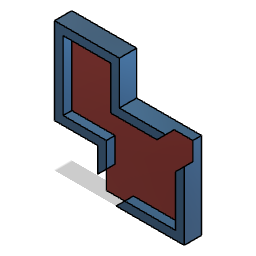
3d07 v122 (Autodesk Fusion 360 design; units mm, degrees)
Autodesk Fusion 360 part; units mm, degrees
sketch "Sketch1" plane through (0, 0, 0) normal (0, 0, 1) x (1, 0, 0)
  line L0 (0, 0) -> (40, 0)
  line L1 (40, 0) -> (40, 40)
  line L2 (40, 40) -> (10, 40)
  line L3 (0, 20) -> (0, 0)
  line L4 (-20, 60) -> (10, 60)
  line L5 (10, 60) -> (10, 40)
  line L6 (0, 20) -> (-20, 20)
  line L7 (-20, 20) -> (-20, 60)
  dimension "d1" = 40
  dimension "d3" = 30
  dimension "d4" = 40
  dimension "d5" = 30
  dimension "d6" = 20
  constraint horizontal L0
  constraint vertical L1
  constraint horizontal L2
  constraint vertical L3
  constraint coincident L0.start L3.end
  constraint horizontal L4
  constraint vertical L5
  constraint horizontal L6
  constraint vertical L7
  measures "d1" distance of L0.start L0.end
  measures "d3" distance of L4.start L4.end
  measures "d4" distance of L4.start L6.end
  measures "d5" distance of L1 L5
  measures "d6" distance of L0 L6
extrude "Extrude1" add sketch "Sketch1" along normal mid plane 4
sketch "Sketch2" plane through (0, 0, 2) normal (0, 0, 1) x (1, 0, 0)
  line L0 (0, 20) -> (0, 0)
  line L1 (0, 0) -> (40, 0)
  line L2 (40, 0) -> (40, 40)
  line L3 (40, 40) -> (10, 40)
  line L4 (10, 40) -> (10, 60)
  line L5 (10, 60) -> (-20, 60)
  line L6 (-20, 60) -> (-20, 20)
  line L7 (-20, 20) -> (0, 20)
  line L8 (-16, 56) -> (6, 56)
  line L9 (6, 56) -> (6, 36)
  line L10 (4, 24) -> (-16, 24)
  line L11 (-16, 24) -> (-16, 56)
  line L12 (36, 4) -> (12.5, 4)
  line L13 (31.5, 40.1168) -> (27.3832, 36)
  line L14 (40, 31.5) -> (36, 27.5)
  line L15 (8.5, 0) -> (12.5, 4)
  line L16 (0, 8.5) -> (4, 12.5)
  line L17 (4, 12.5) -> (4, 24)
  line L18 (6, 36) -> (27.3832, 36)
  line L19 (31.5, 40.1168) -> (31.5, 40)
  line L20 (36, 27.5) -> (36, 4)
  dimension "d9" = 22
  dimension "d10" = 32
  dimension "d11" = 4
  dimension "d12" = 4
  dimension "d16" = 4
  dimension "d18" = 8.5
  dimension "d25" = 32
  dimension "d26" = 4
  dimension "d27" = 8.5
  dimension "d28" = 32
  dimension "d29" = 13.2853
  dimension "d30" = 5.6569
  dimension "d31" = 4.1168
  dimension "d32" = 12.0208
  dimension "d33" = 0.0826
  dimension "d34" = 5.6569
  dimension "d35" = 6.0104
  dimension "d36" = 6.0104
  dimension "d37" = 12.0208
  dimension "d38" = 135
  constraint horizontal L8
  constraint vertical L9
  constraint horizontal L10
  constraint vertical L11
  constraint horizontal L18
  constraint horizontal L12
  constraint vertical L19
  constraint coincident L2 L14.start
  constraint coincident L1 L15.start
  constraint coincident L0 L16.start
  constraint coincident L3 L19.end
  measures "d9" distance of L8.start L8.end
  measures "d10" distance of L8.start L10.end
  measures "d11" distance of L4 L9
  measures "d12" distance of L7 L10
  measures "d16" distance of L1 L12
  measures "d18" distance of L2.end L19
  measures "d25" distance of L17 L20
  measures "d26" distance of L0.end L17
  measures "d27" distance of L0.end L16.start
  measures "d28" distance of L12 L18
  measures "d29" distance of L19.end L14.end
  measures "d30" distance of L14.start L14.end
  measures "d31" horizontal distance of L13.start L13.end
  measures "d32" distance of L14 L19.end
  measures "d33" distance of L13 L16
  measures "d34" distance of L14.start L14.end
  measures "d35" distance of L0.end L15
  measures "d36" distance of L0.end L15
  measures "d37" distance of L15 L16
  measures "d38" angle of L12 L15
extrude "Extrude2" add sketch "Sketch2" along normal blind 4 contours L0 L3 L4 L5 L6 L7 L8 L9 L10 L11 L13 L16 L17 L18 | L1 L2 L12 L14 L15 L20
